Autodesk Fusion 360 part; units mm, degrees
(part 2 of 2)
sketch "Pocket 5 sketch" plane through (0, 0, 0) normal (0, 0, 1) x (1, 0, 0) in component "Dropper plate"
  line L0 (12.335, 1.4172) -> (25.858, 5.0407)
  line L1 (25.858, 5.0407) -> (22.2345, 18.5636)
  line L2 (22.2345, 18.5636) -> (8.7115, 14.9402)
  line L3 (8.7115, 14.9402) -> (12.335, 1.4172)
extrude "Pocket 5" cut sketch "Pocket 5 sketch" along normal blind 14 from surface at 89 bodies 49 in component "Dropper plate"
sketch "Pocket 6 sketch" plane through (0, 0, 0) normal (0, 0, 1) x (1, 0, 0) in component "Dropper plate"
  line L0 (7.2943, 17.3948) -> (17.1938, 27.2943)
  line L1 (17.1938, 27.2943) -> (7.2943, 37.1938)
  line L2 (7.2943, 37.1938) -> (-2.6052, 27.2943)
  line L3 (-2.6052, 27.2943) -> (7.2943, 17.3948)
extrude "Pocket 6" cut sketch "Pocket 6 sketch" along normal blind 14 from surface at 89 bodies 49 in component "Dropper plate"
sketch "Pocket 7 sketch" plane through (0, 0, 0) normal (0, 0, 1) x (1, 0, 0) in component "Dropper plate"
  line L0 (-5.0598, 28.7115) -> (-1.4364, 42.2345)
  line L1 (-1.4364, 42.2345) -> (-14.9593, 45.858)
  line L2 (-14.9593, 45.858) -> (-18.5828, 32.335)
  line L3 (-18.5828, 32.335) -> (-5.0598, 28.7115)
extrude "Pocket 7" cut sketch "Pocket 7 sketch" along normal blind 14 from surface at 89 bodies 49 in component "Dropper plate"
sketch "Pocket 8 sketch" plane through (0, 0, 0) normal (0, 0, 1) x (1, 0, 0) in component "Dropper plate"
  line L0 (-21.4172, 32.335) -> (-25.0407, 45.858)
  line L1 (-25.0407, 45.858) -> (-38.5636, 42.2345)
  line L2 (-38.5636, 42.2345) -> (-34.9402, 28.7115)
  line L3 (-34.9402, 28.7115) -> (-21.4172, 32.335)
extrude "Pocket 8" cut sketch "Pocket 8 sketch" along normal blind 14 from surface at 89 bodies 49 in component "Dropper plate"
sketch "Shaft bore sketch (3)" plane through (0, 0, 0) normal (0, 0, 1) x (1, 0, 0) in component "Dropper plate"
  circle A0 centre (-20, 0) radius 1.5
extrude "Shaft bore''" cut sketch "Shaft bore sketch (3)" along normal blind 14 from surface at 89 bodies 49 in component "Dropper plate"
sketch "N20 gearmotor with encoder sketch" plane through (0, 0, 0) normal (0, 0, 1) x (1, 0, 0) in component "N20 motor"
  line L0 (-25, -6) -> (-15, -6)
  line L1 (-15, -6) -> (-15, 6)
  line L2 (-15, 6) -> (-25, 6)
  line L3 (-25, 6) -> (-25, -6)
extrude "N20 gearmotor with encoder" add sketch "N20 gearmotor with encoder sketch" along normal blind 41.5 from surface at 45.5 separate body makes body 50 in component "N20 motor"
sketch "N20 shaft sketch" plane through (0, 0, 0) normal (0, 0, 1) x (1, 0, 0) in component "N20 motor"
  circle A0 centre (-20, 0) radius 1.5
extrude "N20 shaft" add sketch "N20 shaft sketch" along normal blind 11 from surface at 87 separate body makes body 51 in component "N20 motor"
sketch "Kit 1 sketch" plane through (0, 0, 0) normal (0, 0, 1) x (1, 0, 0) in component "Kits"
  line L0 (-33.632, -30.9773) -> (-36.2979, -40.9263)
  line L1 (-36.2979, -40.9263) -> (-26.3488, -43.5922)
  line L2 (-26.3488, -43.5922) -> (-23.683, -33.6431)
  line L3 (-23.683, -33.6431) -> (-33.632, -30.9773)
extrude "Kit 1" add sketch "Kit 1 sketch" along normal blind 10.3 from surface at 90 separate body makes body 52 in component "Kits"
sketch "Kit 2 sketch" plane through (0, 0, 0) normal (0, 0, 1) x (1, 0, 0) in component "Kits"
  line L0 (-16.317, -33.6431) -> (-13.6512, -43.5922)
  line L1 (-13.6512, -43.5922) -> (-3.7021, -40.9263)
  line L2 (-3.7021, -40.9263) -> (-6.368, -30.9773)
  line L3 (-6.368, -30.9773) -> (-16.317, -33.6431)
extrude "Kit 2" add sketch "Kit 2 sketch" along normal blind 10.3 from surface at 90 separate body makes body 53 in component "Kits"
sketch "Kit 3 sketch" plane through (0, 0, 0) normal (0, 0, 1) x (1, 0, 0) in component "Kits"
  line L0 (0.0111, -27.2943) -> (7.2943, -34.5775)
  line L1 (7.2943, -34.5775) -> (14.5775, -27.2943)
  line L2 (14.5775, -27.2943) -> (7.2943, -20.0111)
  line L3 (7.2943, -20.0111) -> (0.0111, -27.2943)
extrude "Kit 3" add sketch "Kit 3 sketch" along normal blind 10.3 from surface at 90 separate body makes body 54 in component "Kits"
sketch "Kit 4 sketch" plane through (0, 0, 0) normal (0, 0, 1) x (1, 0, 0) in component "Kits"
  line L0 (10.9773, -13.632) -> (20.9263, -16.2979)
  line L1 (20.9263, -16.2979) -> (23.5922, -6.3488)
  line L2 (23.5922, -6.3488) -> (13.6431, -3.683)
  line L3 (13.6431, -3.683) -> (10.9773, -13.632)
extrude "Kit 4" add sketch "Kit 4 sketch" along normal blind 10.3 from surface at 90 separate body makes body 55 in component "Kits"
sketch "Kit 5 sketch" plane through (0, 0, 0) normal (0, 0, 1) x (1, 0, 0) in component "Kits"
  line L0 (13.6431, 3.683) -> (23.5922, 6.3488)
  line L1 (23.5922, 6.3488) -> (20.9263, 16.2979)
  line L2 (20.9263, 16.2979) -> (10.9773, 13.632)
  line L3 (10.9773, 13.632) -> (13.6431, 3.683)
extrude "Kit 5" add sketch "Kit 5 sketch" along normal blind 10.3 from surface at 90 separate body makes body 56 in component "Kits"
sketch "Kit 6 sketch" plane through (0, 0, 0) normal (0, 0, 1) x (1, 0, 0) in component "Kits"
  line L0 (7.2943, 20.0111) -> (14.5775, 27.2943)
  line L1 (14.5775, 27.2943) -> (7.2943, 34.5775)
  line L2 (7.2943, 34.5775) -> (0.0111, 27.2943)
  line L3 (0.0111, 27.2943) -> (7.2943, 20.0111)
extrude "Kit 6" add sketch "Kit 6 sketch" along normal blind 10.3 from surface at 90 separate body makes body 57 in component "Kits"
sketch "Kit 7 sketch" plane through (0, 0, 0) normal (0, 0, 1) x (1, 0, 0) in component "Kits"
  line L0 (-6.368, 30.9773) -> (-3.7021, 40.9263)
  line L1 (-3.7021, 40.9263) -> (-13.6512, 43.5922)
  line L2 (-13.6512, 43.5922) -> (-16.317, 33.6431)
  line L3 (-16.317, 33.6431) -> (-6.368, 30.9773)
extrude "Kit 7" add sketch "Kit 7 sketch" along normal blind 10.3 from surface at 90 separate body makes body 58 in component "Kits"
sketch "Kit 8 sketch" plane through (0, 0, 0) normal (0, 0, 1) x (1, 0, 0) in component "Kits"
  line L0 (-23.683, 33.6431) -> (-26.3488, 43.5922)
  line L1 (-26.3488, 43.5922) -> (-36.2979, 40.9263)
  line L2 (-36.2979, 40.9263) -> (-33.632, 30.9773)
  line L3 (-33.632, 30.9773) -> (-23.683, 33.6431)
extrude "Kit 8" add sketch "Kit 8 sketch" along normal blind 10.3 from surface at 90 separate body makes body 59 in component "Kits"
sketch "Chute tube B left sketch" plane through (0, 0, 0) normal (0, 0, 1) x (1, 0, 0) in component "Chute B left"
  circle A0 centre (0, 0) radius 9
extrude "Chute tube B left" add sketch "Chute tube B left sketch" along normal blind 79.4275 separate body makes body 60 in component "Chute B left"
move_body "Move1'" bodies 60 to x (-0.977496, -0.210954, 0) y (-0.120664, 0.559121, 0.820259) z (-0.173037, 0.801799, -0.571993) at (-47.2943, 27.2943, 79.5) in component "Chute B left"
sketch "Chute bore tool sketch" plane through (0, 0, 0) normal (0, 0, 1) x (1, 0, 0) in component "Chute B left"
  circle A0 centre (0, 0) radius 7.5
extrude "Chute bore tool" add sketch "Chute bore tool sketch" along normal blind 81.4275 separate body makes body 61 in component "Chute B left"
move_body "Move2'" bodies 61 to x (-0.977496, -0.210954, 0) y (-0.120664, 0.559121, 0.820259) z (-0.173037, 0.801799, -0.571993) at (-47.1213, 26.4925, 80.072) in component "Chute B left"
combine "Combine1'" operation cut target body 60 tool bodies 61 in component "Chute B left"
sketch "Exit trim tool sketch" plane through (0, 0, 0) normal (0, 0, 1) x (1, 0, 0) in component "Chute B left"
  circle A0 centre (0, 0) radius 140
  circle A1 centre (0, 0) radius 105
extrude "Exit trim tool" add sketch "Exit trim tool sketch" along normal blind 90 separate body makes body 62 in component "Chute B left"
combine "Combine2'" operation cut target body 60 tool bodies 62 in component "Chute B left"
sketch "Chute tube A right sketch" plane through (0, 0, 0) normal (0, 0, 1) x (1, 0, 0) in component "Chute A right"
  circle A0 centre (0, 0) radius 9
extrude "Chute tube A right" add sketch "Chute tube A right sketch" along normal blind 79.4275 separate body makes body 63 in component "Chute A right"
move_body "Move1''" bodies 63 to x (0.977496, -0.210954, 0) y (-0.120664, -0.559121, 0.820259) z (-0.173037, -0.801799, -0.571993) at (-47.2943, -27.2943, 79.5) in component "Chute A right"
sketch "Chute bore tool sketch (2)" plane through (0, 0, 0) normal (0, 0, 1) x (1, 0, 0) in component "Chute A right"
  circle A0 centre (0, 0) radius 7.5
extrude "Chute bore tool'" add sketch "Chute bore tool sketch (2)" along normal blind 81.4275 separate body makes body 64 in component "Chute A right"
move_body "Move2''" bodies 64 to x (0.977496, -0.210954, 0) y (-0.120664, -0.559121, 0.820259) z (-0.173037, -0.801799, -0.571993) at (-47.1213, -26.4925, 80.072) in component "Chute A right"
combine "Combine1''" operation cut target body 63 tool bodies 64 in component "Chute A right"
sketch "Exit trim tool sketch (2)" plane through (0, 0, 0) normal (0, 0, 1) x (1, 0, 0) in component "Chute A right"
  circle A0 centre (0, 0) radius 140
  circle A1 centre (0, 0) radius 105
extrude "Exit trim tool'" add sketch "Exit trim tool sketch (2)" along normal blind 90 separate body makes body 65 in component "Chute A right"
combine "Combine2''" operation cut target body 63 tool bodies 65 in component "Chute A right"
sketch "GIGA board sketch" plane through (0, 0, 0) normal (0, 0, 1) x (1, 0, 0) in component "Arduino GIGA R1"
  line L0 (-27.56, -66.97) -> (73.96, -66.97)
  line L1 (73.96, -66.97) -> (73.96, -13.63)
  line L2 (73.96, -13.63) -> (-27.56, -13.63)
  line L3 (-27.56, -13.63) -> (-27.56, -66.97)
extrude "GIGA board" add sketch "GIGA board sketch" along normal blind 1.6 from surface at 61.5 separate body makes body 66 in component "Arduino GIGA R1"
sketch "Header strip +y sketch" plane through (0, 0, 0) normal (0, 0, 1) x (1, 0, 0) in component "Arduino GIGA R1"
  line L0 (-23.56, -17.38) -> (69.96, -17.38)
  line L1 (69.96, -17.38) -> (69.96, -14.88)
  line L2 (69.96, -14.88) -> (-23.56, -14.88)
  line L3 (-23.56, -14.88) -> (-23.56, -17.38)
extrude "Header strip +y" add sketch "Header strip +y sketch" along normal blind 8.5 from surface at 63.1 separate body makes body 67 in component "Arduino GIGA R1"
sketch "Header strip -y sketch" plane through (0, 0, 0) normal (0, 0, 1) x (1, 0, 0) in component "Arduino GIGA R1"
  line L0 (-23.56, -65.72) -> (69.96, -65.72)
  line L1 (69.96, -65.72) -> (69.96, -63.22)
  line L2 (69.96, -63.22) -> (-23.56, -63.22)
  line L3 (-23.56, -63.22) -> (-23.56, -65.72)
extrude "Header strip -y" add sketch "Header strip -y sketch" along normal blind 8.5 from surface at 63.1 separate body makes body 68 in component "Arduino GIGA R1"
sketch "Main PCB shield (placeholder) sketch" plane through (0, 0, 0) normal (0, 0, 1) x (1, 0, 0) in component "Main PCB"
  line L0 (-27.56, -66.97) -> (73.96, -66.97)
  line L1 (73.96, -66.97) -> (73.96, -13.63)
  line L2 (73.96, -13.63) -> (-27.56, -13.63)
  line L3 (-27.56, -13.63) -> (-27.56, -66.97)
extrude "Main PCB shield (placeholder)" add sketch "Main PCB shield (placeholder) sketch" along normal blind 1.6 from surface at 71.6 separate body makes body 69 in component "Main PCB"
sketch "PCB component envelope (placeholder) sketch" plane through (0, 0, 0) normal (0, 0, 1) x (1, 0, 0) in component "Main PCB"
  line L0 (-24.56, -63.97) -> (70.96, -63.97)
  line L1 (70.96, -63.97) -> (70.96, -16.63)
  line L2 (70.96, -16.63) -> (-24.56, -16.63)
  line L3 (-24.56, -16.63) -> (-24.56, -63.97)
extrude "PCB component envelope (placeholder)" add sketch "PCB component envelope (placeholder) sketch" along normal blind 7.3 from surface at 73.2 separate body makes body 70 in component "Main PCB"
sketch "Battery (placeholder 7.0 x 3.5 x 2.5) sketch" plane through (0, 0, 0) normal (0, 0, 1) x (1, 0, 0) in component "Battery"
  line L0 (7.5706, 20.1882) -> (76.5071, 32.3436)
  line L1 (76.5071, 32.3436) -> (70.4294, 66.8118)
  line L2 (70.4294, 66.8118) -> (1.4929, 54.6564)
  line L3 (1.4929, 54.6564) -> (7.5706, 20.1882)
extrude "Battery (placeholder 7.0 x 3.5 x 2.5)" add sketch "Battery (placeholder 7.0 x 3.5 x 2.5) sketch" along normal blind 25 from surface at 51 separate body makes body 71 in component "Battery"
sketch "Floor sensor FP (black, blue, red) sketch" plane through (0, 0, 0) normal (0, 0, 1) x (1, 0, 0) in component "Floor port FP"
  line L0 (57, 22) -> (73, 22)
  line L1 (73, 22) -> (73, 38)
  line L2 (73, 38) -> (57, 38)
  line L3 (57, 38) -> (57, 22)
extrude "Floor sensor FP (black, blue, red)" add sketch "Floor sensor FP (black, blue, red) sketch" along normal blind 14 from surface at 28 separate body makes body 72 in component "Floor port FP"
sketch "Silver module SM (straight + 20 deg tilted pair) sketch" plane through (0, 0, 0) normal (0, 0, 1) x (1, 0, 0) in component "Silver module SM"
  line L0 (-10, -11) -> (10, -11)
  line L1 (10, -11) -> (10, 11)
  line L2 (10, 11) -> (-10, 11)
  line L3 (-10, 11) -> (-10, -11)
extrude "Silver module SM (straight + 20 deg tilted pair)" add sketch "Silver module SM (straight + 20 deg tilted pair) sketch" along normal blind 14 from surface at 28 separate body makes body 73 in component "Silver module SM"
component "Chassis" placed x (1, 0, 0) y (0, 1, 0) z (0, 0, 1) at (0, 0, 0)
component "Wheel L" placed x (1, 0, 0) y (0, 1, 0) z (0, 0, 1) at (0, 0, 0)
component "Motor L" placed x (1, 0, 0) y (0, 1, 0) z (0, 0, 1) at (0, 0, 0)
component "Wheel R" placed x (1, 0, 0) y (0, 1, 0) z (0, 0, 1) at (0, 0, 0)
component "Motor R" placed x (1, 0, 0) y (0, 1, 0) z (0, 0, 1) at (0, 0, 0)
component "Omni wheel" placed x (1, 0, 0) y (0, 1, 0) z (0, 0, 1) at (0, 0, 0)
component "Omni arm" placed x (1, 0, 0) y (0, 1, 0) z (0, 0, 1) at (0, 0, 0)
component "Omni pins" placed x (1, 0, 0) y (0, 1, 0) z (0, 0, 1) at (0, 0, 0)
component "Rear nub" placed x (1, 0, 0) y (0, 1, 0) z (0, 0, 1) at (0, 0, 0)
component "Bumper L" placed x (1, 0, 0) y (0, 1, 0) z (0, 0, 1) at (0, 0, 0)
component "Bumper switch L" placed x (1, 0, 0) y (0, 1, 0) z (0, 0, 1) at (0, 0, 0)
component "Bumper R" placed x (1, 0, 0) y (0, 1, 0) z (0, 0, 1) at (0, 0, 0)
component "Bumper switch R" placed x (1, 0, 0) y (0, 1, 0) z (0, 0, 1) at (0, 0, 0)
component "ToF ring" placed x (1, 0, 0) y (0, 1, 0) z (0, 0, 1) at (0, 0, 0)
component "ToF F" placed x (1, 0, 0) y (0, 1, 0) z (0, 0, 1) at (0, 0, 0)
component "ToF FL" placed x (1, 0, 0) y (0, 1, 0) z (0, 0, 1) at (0, 0, 0)
component "ToF FR" placed x (1, 0, 0) y (0, 1, 0) z (0, 0, 1) at (0, 0, 0)
component "ToF SFL" placed x (1, 0, 0) y (0, 1, 0) z (0, 0, 1) at (0, 0, 0)
component "ToF SFR" placed x (1, 0, 0) y (0, 1, 0) z (0, 0, 1) at (0, 0, 0)
component "ToF SRL" placed x (1, 0, 0) y (0, 1, 0) z (0, 0, 1) at (0, 0, 0)
component "ToF SRR" placed x (1, 0, 0) y (0, 1, 0) z (0, 0, 1) at (0, 0, 0)
component "ToF RL" placed x (1, 0, 0) y (0, 1, 0) z (0, 0, 1) at (0, 0, 0)
component "ToF RR" placed x (1, 0, 0) y (0, 1, 0) z (0, 0, 1) at (0, 0, 0)
component "Camera L" placed x (1, 0, 0) y (0, 0.34202, 0.939693) z (0, -0.939693, 0.34202) at (3.0712, 87.9464, 93)
component "Camera R" placed x (-1, 0, 0) y (0, -0.34202, 0.939693) z (0, 0.939693, 0.34202) at (3.0712, -87.9464, 93)
component "Lid" placed x (1, 0, 0) y (0, 1, 0) z (0, 0, 1) at (0, 0, 0)
component "Start button" placed x (1, 0, 0) y (0, 1, 0) z (0, 0, 1) at (0, 0, 0)
component "Victim LED" placed x (1, 0, 0) y (0, 1, 0) z (0, 0, 1) at (0, 0, 0)
component "Dropper floor" placed x (1, 0, 0) y (0, 1, 0) z (0, 0, 1) at (0, 0, 0)
component "Dropper plate" placed x (1, 0, 0) y (0, 1, 0) z (0, 0, 1) at (0, 0, 0)
component "N20 motor" placed x (1, 0, 0) y (0, 1, 0) z (0, 0, 1) at (0, 0, 0)
component "Kits" placed x (1, 0, 0) y (0, 1, 0) z (0, 0, 1) at (0, 0, 0)
component "Chute B left" placed x (1, 0, 0) y (0, 1, 0) z (0, 0, 1) at (0, 0, 0)
component "Chute A right" placed x (1, 0, 0) y (0, 1, 0) z (0, 0, 1) at (0, 0, 0)
component "Arduino GIGA R1" placed x (1, 0, 0) y (0, 1, 0) z (0, 0, 1) at (0, 0, 0)
component "Main PCB" placed x (1, 0, 0) y (0, 1, 0) z (0, 0, 1) at (0, 0, 0)
component "Battery" placed x (1, 0, 0) y (0, 1, 0) z (0, 0, 1) at (0, 0, 0)
component "Floor port FP" placed x (1, 0, 0) y (0, 1, 0) z (0, 0, 1) at (0, 0, 0)
component "Silver module SM" placed x (1, 0, 0) y (0, 1, 0) z (0, 0, 1) at (0, 0, 0)
named bodies: "Chassis shell", "Chute hole tool B left", "Chute hole tool A right", "Wheel L", "Encoder L", "Gearmotor L", "Motor shaft L", "Wheel R", "Encoder R", "Gearmotor R", "Motor shaft R", "Omni wheel", "Arm plate L", "Arm plate R", "Pivot pin", "Axle pin", "Rear nub", "Bumper plate L", "Microswitch L", "Bumper plate R", "Microswitch R", "ToF ring", "VL53L0X module F", "VL53L0X chip F", "VL53L0X module FL", "VL53L0X chip FL", "VL53L0X module FR", "VL53L0X chip FR", "VL53L0X module SFL", "VL53L0X chip SFL", "VL53L0X module SFR", "VL53L0X chip SFR", "VL53L0X module SRL", "VL53L0X chip SRL", "VL53L0X module SRR", "VL53L0X chip SRR", "VL53L0X module RL", "VL53L0X chip RL", "VL53L0X module RR", "VL53L0X chip RR", "Lens block L", "OpenMV H7 Plus board L", "Lens block R", "OpenMV H7 Plus board R", "Lid", "Start button", "Victim LED", "Dropper floor", "Dropper plate", "N20 gearmotor with encoder", "N20 shaft", "Kit 1", "Kit 2", "Kit 3", "Kit 4", "Kit 5", "Kit 6", "Kit 7", "Kit 8", "Chute tube B left", "Chute bore tool", "Exit trim tool", "Chute tube A right", "GIGA board", "Header strip +y", "Header strip -y", "Main PCB shield (placeholder)", "PCB component envelope (placeholder)", "Battery (placeholder 7.0 x 3.5 x 2.5)", "Floor sensor FP (black, blue, red)", "Silver module SM (straight + 20 deg tilted pair)"
